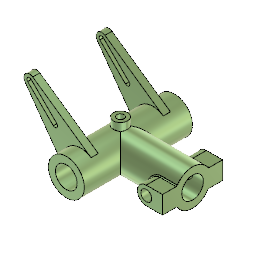
mechanical linkage component (Autodesk Fusion 360 design; units mm, degrees)
Autodesk Fusion 360 part; units mm, degrees
note: some values were not read from the file. Set by a fixed rule: which sketch regions a step uses.
sketch "Sketch1" plane through (0, 0, 0) normal (0, 1, 0) x (1, 0, 0)
  circle A0 centre (0, 0) radius 25
  circle A1 centre (0, 0) radius 15
  line L0 (0, 0) -> (-71.0563, -70.3634) construction
  circle A2 centre (-71.0563, -70.3634) radius 8
  line L1 (-77.5698, -65.7186) -> (-20.3547, 14.515)
  line L2 (-66.4755, -76.9221) -> (14.3149, -20.4959)
  line L3 (-68.5935, -72.8504) -> (-33.0654, -37.6687)
  arc A3 (-33.0654, -37.6687) -> (-37.9908, -32.6947) centre (-35.5281, -35.1817) ccw
  line L4 (-37.9908, -32.6947) -> (-73.519, -67.8764)
  arc A4 (-73.519, -67.8764) -> (-68.5935, -72.8504) centre (-71.0563, -70.3634) ccw
  line L5 (-71.0563, -70.3634) -> (-35.5281, -35.1817) construction
  line L6 (0, 0) -> (100, 0) construction
  dimension "d1" = 50
  dimension "d2" = 30
  dimension "d3" = 100
  dimension "d4" = 16
  dimension "d5" = 7
  dimension "d6" = 100
  constraint coincident A0.centre A1.centre
  constraint coincident L0.end A2.centre
  constraint coincident A2 L1.start
  constraint coincident A0 L1.end
  constraint tangent A0 L1
  constraint coincident A2 L2.start
  constraint coincident A0 L2.end
  constraint tangent A0 L2
  constraint tangent A2 L1
  constraint tangent A2 L2
  constraint tangent L3 A3
  constraint tangent A3 L4
  constraint parallel L3 L4
  constraint tangent L4 A4
  constraint tangent L3 A4
  constraint parallel L0 L5
  constraint horizontal L6
  measures "d1" diameter of A0
  measures "d2" diameter of A1
  measures "d3" distance of A0.centre L0.end
  measures "d4" diameter of A2
  measures "d5" diameter of A3
  measures "d6" distance of A0.centre L6.end
extrude "Extrude1" add sketch "Sketch1" along normal mid plane 150 contours A0
extrude "Extrude2" add sketch "Sketch1" along normal blind 10 from surface at 45 contours A0 A2 L1 L2 L3 A3 L4 | A2 L3 L4 A4 picked at (-76.6312, -67.0523)
mirror "Mirror1" about plane through (0, 0, 0) normal (0, 1, 0) of "Extrude2"
sketch "Sketch2" plane through (0, 0, 0) normal (1, 0, 0) x (0, 1, 0)
  line L0 (-45, 65.7186) -> (-45, 25)
  line L1 (-55, 25) -> (-55, 65.7186)
  line L2 (-45, 65.7186) -> (-45, 78.3634)
  line L3 (-55, 65.7186) -> (-55, 78.3634)
  line L4 (-75, 0) -> (-75, -25)
  line L5 (-75, 25) -> (-75, 0)
  line L6 (75, 0) -> (75, 25)
  line L7 (75, -25) -> (75, 0)
  line L8 (45, 65.7186) -> (45, 25)
  line L9 (55, 25) -> (55, 65.7186)
  line L10 (45, 65.7186) -> (45, 78.3634)
  line L11 (55, 65.7186) -> (55, 78.3634)
  line L12 (-55, 78.3634) -> (-45, 78.3634)
  line L13 (-75, -25) -> (75, -25)
  line L14 (-75, 25) -> (-55, 25)
  line L15 (-45, 25) -> (45, 25)
  line L16 (55, 25) -> (75, 25)
  line L17 (45, 78.3634) -> (55, 78.3634)
  circle A0 centre (0, 0) radius 25
  circle A1 centre (0, 0) radius 15
  line L18 (-41.7186, 12.5) -> (-41.7186, -12.5)
  line L19 (-41.7186, -12.5) -> (-21.6506, -12.5)
  line L20 (-41.7186, 12.5) -> (-21.6506, 12.5)
  dimension "d14" = 50
  dimension "d15" = 30
  dimension "d16" = 25
  dimension "d17" = 12.5
  constraint coincident A0.centre A1.centre
  constraint concentric A0 A1
  constraint vertical L18
  constraint coincident A0 L19.end
  constraint perpendicular L18 L19
  constraint coincident A0 L20.end
  constraint perpendicular L18 L20
  measures "d14" diameter of A0
  measures "d15" diameter of A1
  measures "d16" distance of L18.start L18.end
  measures "d17" vertical distance of A0.centre L18.start
extrude "Extrude3" add sketch "Sketch2" along normal blind 100 contours A0
extrude "Extrude4" cut sketch "Sketch1" along normal mid plane 200 contours A1
extrude "Extrude5" cut sketch "Sketch2" along normal blind 140 contours A1
extrude "Extrude6" add sketch "Sketch2" against normal blind 35 from surface at 100 contours A0 L18 L19 L20
mirror "Mirror2" about plane through (0, 0, 0) normal (0, 1, 0) of "Extrude6"
fillet "Fillet1" radius 12.5 4 edges at (65, -31.6846, 12.5) (65, 31.6846, 12.5) (65, 31.6846, -12.5) (65, -31.6846, -12.5)
fillet "Fillet2" radius 2 8 edges at (88.75, -21.6506, -12.5) (68.6701, -23.382, -8.8478) (68.6701, -23.382, 8.8478) (88.75, -21.6506, 12.5) (88.75, 21.6506, 12.5) (68.6701, 23.382, 8.8478) (68.6701, 23.382, -8.8478) (88.75, 21.6506, -12.5)
hole "Hole1" at (77.5, -41.7186, 0) direction (0, 1, 0) diameter 15 end through all
ref_plane "WorkPlane1" through (0, 0, 35) normal (0, 0, 1) x (1, 0, 0)
sketch "Sketch3" plane through (0, 0, 35) normal (0, 0, 1) x (1, 0, 0)
  circle A0 centre (0, 0) radius 10
  circle A1 centre (0, 0) radius 5
  dimension "d36" = 20
  dimension "d37" = 10
  constraint coincident A0.centre A1.centre
  constraint concentric A0 A1
  measures "d36" diameter of A0
  measures "d37" diameter of A1
extrude "Extrude7" add sketch "Sketch3" against normal blind 15
extrude "Extrude8" cut sketch "Sketch3" against normal blind 25 contours A1
